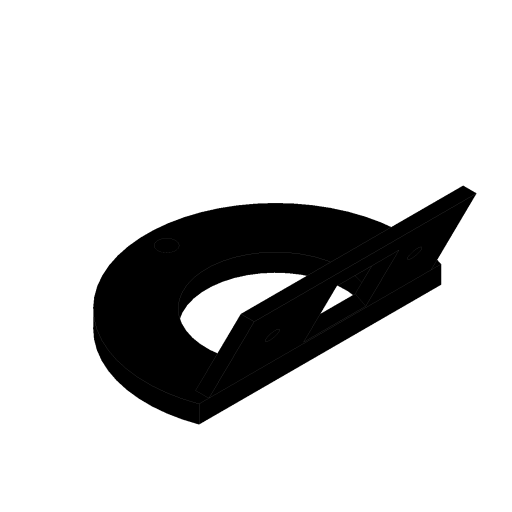
# Autodesk Inventor part: Nose cam retention
Saved by Autodesk Inventor 2024 (Build 280153000, 153)
## iProperties
Created: 2024-03-27
Part Number: Nose cam retention
Material: Generic
Document SubType Name: Modeling
Designer: Maur
Density: 1 g/cm^3
Appearance: Default
Author: Maur
Autodesk Inventor part; units mm, degrees
ref_plane "YZ Plane" through (0, 0, 0) normal (1, 0, 0) x (0, 1, 0)
ref_plane "XZ Plane" through (0, 0, 0) normal (0, 1, 0) x (-1, 0, 0)
ref_plane "XY Plane" through (0, 0, 0) normal (0, 0, 1) x (1, 0, 0)
sketch "Sketch1" plane through (0, 0, 0) normal (0, 1, 0) x (-1, 0, 0)
  circle A0 centre (0, 0) radius 29
  dimension "d0" = 58
  constraints: 1 centre point, 1 coincident
  measures "d0" diameter of A0
extrude "Extrusion1" add sketch "Sketch1" along normal blind 4
sketch "Sketch2" plane through (0, 4, 0) normal (0, 1, 0) x (1, 0, 0)
  circle A0 centre (0, 0) radius 15.5
  dimension "d3" = 31
  constraints: 1 centre point, 1 coincident
  measures "d3" diameter of A0
extrude "Extrusion2" cut sketch "Sketch2" against normal through all
sketch "Sketch3" plane through (0, 4, 0) normal (0, 1, 0) x (1, 0, 0)
  circle A0 centre (-24.5, 0) radius 2
  point P0 (0, 0)
  dimension "d6" = 24.5
  dimension "d7" = 4
  constraints: 1 centre point
  measures "d6" distance of point (0, 0) A0.centre
  measures "d7" diameter of A0
extrude "Extrusion3" cut sketch "Sketch3" against normal through all
sketch "Sketch4" plane through (0, 4, 0) normal (0, 1, 0) x (1, 0, 0)
  line L0 (10, -34.3438) -> (33.4765, -34.3438)
  line L1 (33.4765, -34.3438) -> (33.4765, 39.4177)
  line L2 (33.4765, 39.4177) -> (10, 39.4177)
  line L3 (10, 39.4177) -> (10, -34.3438)
  point P0 (0, 0)
  dimension "d13" = 10
  constraints: 8 end point, 2 parallel, 1 horizontal, 1 perpendicular
  measures "d13" distance from line of point (0, 0) L3
extrude "Extrusion4" cut sketch "Sketch4" against normal blind 10
sketch "Sketch5" plane through (0, 0, 0) normal (0, 0, 1) x (1, 0, 0)
  line L0 (10, 4) -> (-29, 4) projected
  line L1 (10, 4) -> (20.1905, 24)
  line L2 (10, 4) -> (32.4465, 4) construction
  line L3 (20.1905, 24) -> (17.1905, 24)
  line L4 (17.1905, 24) -> (7, 4)
  line L5 (7, 4) -> (10, 4)
  line L6 (10, 0) -> (10, 4) projected
  line L7 (10, 4) -> (10, 0)
  line L8 (7, 4) -> (4.9619, 0)
  line L9 (10, 0) -> (-15.5, 0) projected
  line L10 (4.9619, 0) -> (10, 0)
  point P0 (0, 0)
  point P1 (7, 4)
  point P2 (18.6905, 24)
  dimension "d16" = 63
  dimension "d17" = 3
  dimension "d18" = 117
  dimension "d21" = 20
  constraints: 16 end point, 3 horizontal, 1 equal length, 1 midpoint, 1 parallel, 1 point on line, 1 vertical
  measures "d16" angle of L2 L1
  measures "d17" distance of L1.end L3.end
  measures "d18" angle of L4 L3
  measures "d21" distance from line of L0 point (18.691, 24)
extrude "Extrusion5" add sketch "Sketch5" along normal mid plane 50 contours L0 L4 L3 L1
sketch "Sketch6" plane through (7, 4, -25) normal (-0.891, 0.454, 0) x (0, 0, 1)
  line L0 (11.1707, 0) -> (38.8293, 0) projected
  line L1 (15, 2) -> (29, 2)
  line L2 (29, 2) -> (29, 18.4465)
  line L3 (29, 18.4465) -> (15, 18.4465)
  line L4 (15, 18.4465) -> (15, 2)
  line L5 (50, 22.4465) -> (0, 22.4465) projected
  point P0 (25, -6.742)
  point P1 (25, 0)
  point P2 (25, 0)
  point P3 (40, 22.4465)
  point P4 (10, 22.4465)
  dimension "d37" = 4
  dimension "d38" = 10
  dimension "d39" = 4
  dimension "d40" = 2
  constraints: 8 end point, 2 midpoint, 2 parallel, 1 horizontal, 1 perpendicular
  measures "d37" distance from line of point (25, 0) L2
  measures "d38" distance from line of point (25, 0) L4
  measures "d39" distance between parallel lines of L5 L3
  measures "d40" distance between parallel lines of L0 L1
extrude "Extrusion6" cut sketch "Sketch6" against normal blind 46
sketch "Sketch7" plane through (7, 4, -25) normal (-0.891, 0.454, 0) x (0, 0, 1)
  circle A0 centre (9, 13) radius 1.5
  circle A1 centre (41, 13) radius 1.5
  line L0 (50, 0) -> (38.8293, 0) projected
  line L1 (11.1707, 0) -> (0, 0) projected
  ellipse E0 centre (25, -14.3007) end of major axis (27, -14.3007) minor radius 0.908 projected
  point P0 (25, -6.742)
  dimension "d29" = 3
  dimension "d30" = 3
  dimension "d31" = 13
  dimension "d32" = 13
  dimension "d46" = 16
  dimension "d47" = 16
  constraints: 2 centre point
  measures "d29" diameter of A0
  measures "d30" diameter of A1
  measures "d31" distance from line of L0 A1.centre
  measures "d32" distance from line of L1 A0.centre
  measures "d46" horizontal distance of E0.centre A0.centre
  measures "d47" horizontal distance of A1.centre E0.centre
extrude "Extrusion7" cut sketch "Sketch7" against normal blind 46 contours A0 | A1
sketch "Sketch8" plane through (0, 0, 25) normal (0, 0, 1) x (1, 0, 0)
  line L0 (10, 4) -> (10, 0) projected
  line L1 (10, 4) -> (10, 0)
  line L2 (10, 4) -> (-29, 4) projected
  line L3 (7, 4) -> (4.9619, 0)
  line L4 (10, 0) -> (-29, 0) projected
  line L5 (7, 4) -> (11.4893, 4) construction
  line L6 (4.9619, 0) -> (10, 0)
  point P0 (0, 0)
  dimension "d43" = 117
  constraints: 8 end point, 2 point on line, 1 collinear, 1 equal length, 1 horizontal, 1 vertical
  measures "d43" angle of L3 L5
extrude "Extrusion8" add sketch "Sketch8" against normal blind 46
body "Solid1"
